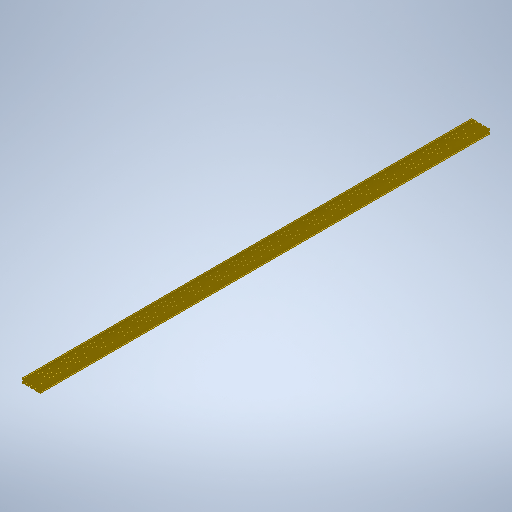
# Autodesk Inventor part: Perfil 20×40 6 rasgos_AST02004006
Saved by Autodesk Inventor 2025.2 (Build 292293000, 293)
## iProperties
Created: 2025-04-02
Part Number: Perfil 20×40 6 rasgos_AST02004006
Material: Ouro
Document SubType Name: Modeling
Designer: Gustavo Sousa
Density: 19.3 g/cm^3
Appearance: Metal quente 2400F
Author: Gustavo Sousa
Autodesk Inventor part; units mm, degrees
ref_plane "YZ Plane" through (0, 0, 0) normal (1, 0, 0) x (0, 1, 0)
ref_plane "XZ Plane" through (0, 0, 0) normal (0, 1, 0) x (-1, 0, 0)
ref_plane "XY Plane" through (0, 0, 0) normal (0, 0, 1) x (1, 0, 0)
sketch "Esboço3" plane through (0, 0, 0) normal (0, 0, 1) x (1, 0, 0)
  line L0 (-40, 10) -> (40, 10) construction
  line L1 (-40, 10) -> (-40, -10) construction
  line L2 (-34, 3.1) -> (-34, -3.1) construction
  circle A0 centre (-30, 0) radius 2.5 construction
  line L3 (-40, 10) -> (-20, 10) construction
  line L4 (-30, 0) -> (-40, 10) construction
  line L5 (-33.1, 4) -> (-26.9, 4) construction
  line L6 (-33.1, 10) -> (-26.9, 10) construction
  arc A1 (-39.5, 10) -> (-40, 9.5) centre (-39.5, 9.5) ccw
  line L7 (-38, 3.1) -> (-38, 7.1) construction
  line L8 (-34, 3.1) -> (-38, 7.1) construction
  line L9 (-40, 3.1) -> (-40, -3.1) construction
  line L10 (-40, 9.5) -> (-40, 3.1) construction
  line L11 (-40, 3.1) -> (-38, 3.1) construction
  line L12 (-33.1, 10) -> (-33.1, 8) construction
  line L13 (-33.1, 8) -> (-37.1, 8) construction
  line L14 (-39.5, 10) -> (-33.1, 10) construction
  line L15 (-37.1, 8) -> (-33.1, 4) construction
  line L16 (-33.1, 10) -> (-33.6, 10) construction
  line L17 (-33.6, 10) -> (-33.6, 9.5)
  line L18 (-33.6, 9.5) -> (-33.1, 9.5)
  line L19 (-33.1, 9.5) -> (-33.1, 10) construction
  arc A2 (-35.8929, 8) -> (-36.2464, 7.1464) centre (-35.8929, 7.5) ccw
  arc A3 (-33.2464, 4.1464) -> (-32.8929, 4) centre (-32.8929, 4.5) ccw
  arc A4 (-27.1071, 4) -> (-26.7536, 4.1464) centre (-27.1071, 4.5) ccw
  arc A5 (-23.7536, 7.1464) -> (-24.1071, 8) centre (-24.1071, 7.5) ccw
  arc A6 (-37.1464, 6.2464) -> (-38, 5.8929) centre (-37.5, 5.8929) ccw
  arc A7 (-34, 2.8929) -> (-34.1464, 3.2464) centre (-34.5, 2.8929) ccw
  line L20 (-40, 3.1) -> (-39.5, 3.1) construction
  line L21 (-39.5, 3.1) -> (-39.5, 3.6)
  line L22 (-39.5, 3.6) -> (-40, 3.6)
  line L23 (-40, 3.6) -> (-40, 3.1) construction
  line L24 (-39.5, 10) -> (-33.6, 10)
  line L25 (-33.1, 9.5) -> (-33.1, 8)
  line L26 (-33.1, 8) -> (-35.8929, 8)
  line L27 (-36.2464, 7.1464) -> (-33.2464, 4.1464)
  line L28 (-40, 9.5) -> (-40, 3.6)
  line L29 (-39.5, 3.1) -> (-38, 3.1)
  line L30 (-38, 3.1) -> (-38, 5.8929)
  line L31 (-37.1464, 6.2464) -> (-34.1464, 3.2464)
  line L32 (-34, 2.8929) -> (-34, 0)
  line L33 (-32.8929, 4) -> (-30, 4)
  line L34 (-30, 4) -> (-26.9, 4) construction
  line L35 (-26.9, 10) -> (-20, 10) construction
  line L36 (-26, 3.1) -> (-26, -3.1) construction
  line L37 (-30, 0) -> (-20, 10) construction
  line L38 (-26.9, 10) -> (-26.4, 10) construction
  line L39 (-26.4, 10) -> (-26.4, 9.5)
  line L40 (-26.4, 9.5) -> (-26.9, 9.5)
  line L41 (-26.9, 9.5) -> (-26.9, 10) construction
  line L42 (-26.9, 10) -> (-26.9, 8) construction
  line L43 (-26.9, 8) -> (-22.9, 8) construction
  line L44 (-26.9, 4) -> (-22.9, 8) construction
  line L45 (-26.9, 9.5) -> (-26.9, 8)
  line L46 (-27.1071, 4) -> (-30, 4)
  line L47 (-26.9, 8) -> (-24.1071, 8)
  line L48 (-23.7536, 7.1464) -> (-26.7536, 4.1464)
  line L49 (-26.4, 10) -> (-20, 10)
  line L50 (-26, 3.1) -> (-20.2313, 8.8687) construction
  line L51 (-20, 10) -> (-20, 9) construction
  arc A8 (-20, 9) -> (-20.2313, 8.8687) centre (-19.8777, 8.5152) ccw
  arc A9 (-25.8536, 3.2464) -> (-26, 2.8929) centre (-25.5, 2.8929) ccw
  line L52 (-26, 2.8929) -> (-26, 0)
  line L53 (-25.8536, 3.2464) -> (-20.2313, 8.8687)
  arc A10 (-30, 2.5) -> (-32.5, 0) centre (-30, 0) ccw
  line L54 (-34, 0) -> (-32.5, 0)
  arc A11 (-27.5, 0) -> (-30, 2.5) centre (-30, 0) ccw
  line L55 (-27.5, 0) -> (-26, 0)
  line L56 (-20, 10) -> (0, 10) construction
  circle A12 centre (-10, 0) radius 2.5 construction
  line L57 (-13.1, 4) -> (-6.9, 4) construction
  line L58 (-14, 3.1) -> (-14, -3.1) construction
  line L59 (-10, 0) -> (-20, 10) construction
  line L60 (-13.1, 10) -> (-6.9, 10) construction
  line L61 (-20, 10) -> (-13.1, 10) construction
  line L62 (-13.1, 10) -> (-13.1, 8) construction
  line L63 (-13.1, 8) -> (-17.1, 8) construction
  line L64 (-17.1, 8) -> (-13.1, 4) construction
  line L65 (-19.7687, 8.8687) -> (-14, 3.1) construction
  arc A13 (-19.7687, 8.8687) -> (-20, 9) centre (-20.1223, 8.5152) ccw
  line L66 (-13.1, 10) -> (-13.6, 10) construction
  line L67 (-13.6, 10) -> (-13.6, 9.5)
  line L68 (-13.6, 9.5) -> (-13.1, 9.5)
  line L69 (-13.1, 9.5) -> (-13.1, 10) construction
  line L70 (-13.1, 9.5) -> (-13.1, 8)
  line L71 (-20, 10) -> (-13.6, 10)
  arc A14 (-15.8929, 8) -> (-16.2464, 7.1464) centre (-15.8929, 7.5) ccw
  arc A15 (-13.2464, 4.1464) -> (-12.8929, 4) centre (-12.8929, 4.5) ccw
  line L72 (-14, 3.1) -> (-14, 0) construction
  arc A16 (-10, 2.5) -> (-12.5, 0) centre (-10, 0) ccw
  line L73 (-14, 0) -> (-12.5, 0)
  line L74 (-10, 0) -> (0, 10) construction
  arc A17 (-7.5, 0) -> (-10, 2.5) centre (-10, 0) ccw
  line L75 (-13.1, 8) -> (-15.8929, 8)
  line L76 (-16.2464, 7.1464) -> (-13.2464, 4.1464)
  line L77 (-6.9, 10) -> (0, 10) construction
  line L78 (-6.9, 10) -> (-6.9, 8) construction
  line L79 (-6.9, 8) -> (-2.9, 8) construction
  line L80 (-6.9, 4) -> (-2.9, 8) construction
  line L81 (-6.9, 10) -> (-6.4, 10) construction
  line L82 (-6.4, 10) -> (-6.4, 9.5)
  line L83 (-6.4, 9.5) -> (-6.9, 9.5)
  line L84 (-6.9, 9.5) -> (-6.9, 10) construction
  arc A18 (-3.7536, 7.1464) -> (-4.1071, 8) centre (-4.1071, 7.5) ccw
  arc A19 (-7.1071, 4) -> (-6.7536, 4.1464) centre (-7.1071, 4.5) ccw
  line L85 (-6.9, 9.5) -> (-6.9, 8)
  line L86 (-6.9, 8) -> (-4.1071, 8)
  line L87 (-3.7536, 7.1464) -> (-6.7536, 4.1464)
  line L88 (-12.8929, 4) -> (-10, 4)
  line L89 (-10, 4) -> (-7.1071, 4)
  line L90 (-6, 3.1) -> (-6, -3.1) construction
  arc A20 (-14, 2.8929) -> (-14.1464, 3.2464) centre (-14.5, 2.8929) ccw
  line L91 (-19.7687, 8.8687) -> (-14.1464, 3.2464)
  line L92 (-14, 2.8929) -> (-14, 0)
  line L93 (-7.5, 0) -> (-6, 0)
  line L94 (-6, 3.1) -> (-0.2313, 8.8687) construction
  line L95 (0, 10) -> (0, 9)
  arc A21 (0, 9) -> (-0.2313, 8.8687) centre (0.1223, 8.5152) ccw
  arc A22 (-5.8536, 3.2464) -> (-6, 2.8929) centre (-5.5, 2.8929) ccw
  line L96 (-5.8536, 3.2464) -> (-0.2313, 8.8687)
  line L97 (-6, 2.8929) -> (-6, 0)
  line L98 (-6.4, 10) -> (0, 10)
  point P0 (0, 0)
  point P1 (-30, 10)
  point P2 (-40, 0)
  point P3 (-40, 0)
  point P4 (-30, 10)
  point P5 (-40, 0)
  point P6 (-10, 10)
  point P7 (-10, 10)
  point P8 (-26.9, 9)
  point P9 (-6.75, 0)
  point P10 (-6.9, 9)
  point P11 (-7.5, 0)
  dimension "d45" = 80
  dimension "d46" = 10
  dimension "d47" = 20
  dimension "d48" = 6.2
  dimension "d49" = 5
  dimension "d51" = 6
  dimension "d54" = 0.5
  dimension "d56" = 2
  dimension "d57" = 0.5
  dimension "d59" = 4
  dimension "d67" = 1.5
  constraints: 198 end point, 49 point on circle, 37 tangent, 28 point on line, 26 collinear, 26 equal length, 24 horizontal, 23 centre point, 18 parallel, 17 equal radius, 17 midpoint, 16 horizontal alignment, 15 vertical, 8 coincident, 7 vertical alignment, 6 perpendicular
  measures "d45" distance of L0.start L0.end
  measures "d46" distance from line of point (0, 0) L0
  measures "d47" distance of L0.start L1.end
  measures "d48" distance of L2.start L2.end
  measures "d49" diameter of A0
  measures "d51" distance between parallel lines of L1 L2
  measures "d54" radius of A1
  measures "d56" distance between parallel lines of L10 L7
  measures "d57" distance of L17.end L18.end
  measures "d59" distance from line of L4.start L36
  measures "d67" distance of L72.end L73.end
extrude "Extrusão3" add sketch "Esboço3" along normal mid plane 2000
mirror "Espelhar7" about plane through (0, 0, 0) normal (0, 1, 0) of "Extrusão3"
mirror "Espelhar8" about plane through (0, 0, 0) normal (1, 0, 0) of "Extrusão3", "Espelhar7"
fillet "Arredondamento5" radius 1 10 edges at (-20, 9, 500) (-20, 9, -500) (0, 9, 0) (20, 9, 500) (20, 9, -500) (-20, -9, 500) (-20, -9, -500) (0, -9, 0) (20, -9, 500) (20, -9, -500)
